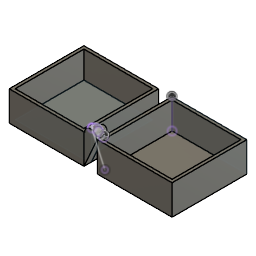
19_20_DAY - Parametric Box (Autodesk Fusion 360 design; units mm, degrees)
part number: 2026-01-02-10-23-45-080
part number: 2026-01-02-10-51-27-139
part number: 2026-01-02-23-14-10-436
Autodesk Fusion 360 part; units mm, degrees
sketch "Box Bottom" plane through (0, 0, 0) normal (0, 1, 0) x (1, 0, 0) in component "Box Top"
  line L0 (0, 0) -> (50, 0)
  line L1 (50, 0) -> (50, 50)
  line L2 (50, 50) -> (0, 50)
  line L3 (0, 50) -> (0, 0)
  dimension "d3" = 50
  dimension "d4" = 50
  constraint horizontal L0
  constraint vertical L1
  constraint horizontal L2
  constraint vertical L3
  constraint coincident L0.start L3.end
  measures "d3" distance of L0.start L2.end
  measures "d4" distance of L1.end L2.end
extrude "Extrude1" add sketch "Box Bottom" along normal blind 20 makes body 1 in component "Box Top"
shell "Shell1" thickness 2 removed faces 1 at (16.6667, 20, -33.3333) on bodies 1 in component "Box Top"
sketch "Box Bottom (2)" plane through (0, 0, 0) normal (0, 1, 0) x (1, 0, 0) in component "Box Top (1)"
  line L0 (0, 0) -> (50, 0)
  line L1 (50, 0) -> (50, 50)
  line L2 (50, 50) -> (0, 50)
  line L3 (0, 50) -> (0, 0)
  dimension "d3_1" = 50
  dimension "d4_1" = 50
  constraint horizontal L0
  constraint vertical L1
  constraint horizontal L2
  constraint vertical L3
  constraint coincident L0.start L3.end
  measures "d3_1" distance of L0.start L2.end
  measures "d4_1" distance of L1.end L2.end
extrude "Extrude1'" add sketch "Box Bottom (2)" along normal blind 20 separate body makes body 2 in component "Box Top (1)"
shell "Shell1'" thickness 2 removed faces 1 at (16.6667, 20, -33.3333) on bodies 2 in component "Box Top (1)"
sketch "Sketch1" plane through (0, 0, 0) normal (0, 0, 1) x (1, 0, 0)
  line L0 (-59, 0) -> (-9, 0)
  line L1 (-9, 0) -> (-9, 20)
  line L2 (-9, 20) -> (-59, 20)
  line L3 (-59, 20) -> (-59, 0)
  line L4 (-9, 20) -> (-4.5, 20)
  circle A0 centre (-4.5, 20) radius 4
  line L5 (-9, 0) -> (-0.8439, 18.3774)
  dimension "d16" = 4.5
  dimension "d17" = 8
  constraint coincident L1.end L2.start
  constraint perpendicular L1 L4
  constraint coincident L4.end A0.centre
  constraint coincident L0.end L1.start
  constraint coincident A0 L5.end
  constraint tangent A0 L5
  measures "d16" distance of L1.end L4.end
  measures "d17" diameter of A0
extrude "Extrude1''" add sketch "Sketch1" against normal blind 5 separate body contours L1 L4 A0 L5 | A0 makes body 3
sketch "Sketch2" plane through (0, 0, -5) normal (0, 0, -1) x (-1, 0, 0)
  line L0 (9, 0) -> (9, 20)
  line L1 (9, 20) -> (8.5, 20)
  arc A0 (8.5, 20) -> (0.8439, 18.3774) centre (4.5, 20) ccw
  line L2 (0.8439, 18.3774) -> (9, 0)
  arc A1 (8.5, 20) -> (0.8439, 18.3774) centre (4.5, 20) ccw
  circle A2 centre (4.5, 20) radius 2
  dimension "d20" = 4
  constraint concentric A1 A2
  measures "d20" diameter of A2
extrude "Extrude2" add sketch "Sketch2" along normal blind 3.8 contours A2 bodies 3
sketch "Sketch3" plane through (0, 2, 0) normal (0, 1, 0) x (-1, 0, 0)
  line L0 (57, -48) -> (57, -2)
  line L1 (57, -2) -> (11, -2)
  line L2 (11, -2) -> (11, -48)
  line L3 (11, -48) -> (57, -48)
sketch "Sketch4" plane through (0, 0, -5) normal (0, 0, -1) x (-1, 0, 0)
  circle A0 centre (4.5, 20) radius 2
  line L0 (9, 0) -> (9, 20)
  line L1 (9, 20) -> (8.5, 20)
  arc A1 (8.5, 20) -> (0.8439, 18.3774) centre (4.5, 20) ccw
  line L2 (0.8439, 18.3774) -> (9, 0)
  arc A2 (8.5, 20) -> (0.8439, 18.3774) centre (4.5, 20) ccw
  circle A3 centre (4.5, 20) radius 4
  line L3 (0, 20) -> (0.5, 20)
  line L4 (0, 0) -> (8.1561, 18.3774)
  constraint concentric A2 A3
  constraint coincident A2 L3.end
  constraint coincident A3 L3.end
  constraint coincident L4.start origin
  constraint coincident A3 L4.end
  constraint tangent A3 L4
  constraint horizontal L3
sketch "Sketch5" plane through (0, 0, -50) normal (0, 0, -1) x (-1, 0, 0)
  line L0 (-50, 0) -> (0, 0)
  line L1 (0, 0) -> (0, 20)
  line L2 (0, 20) -> (-50, 20)
  line L3 (-50, 20) -> (-50, 0)
  line L4 (0, 0) -> (0, 20)
  line L5 (0.5, 20) -> (0, 20)
  constraint coincident L1.end L2.start
  constraint horizontal L5
component "Box Top" placed x (1, 0, 0) y (0, 1, 0) z (0, 0, 1) at (0, 0, 0)
component "Box Top (1)" placed x (1, 0, 0) y (0, 1, 0) z (0, 0, 1) at (-59, 0, 0)
equation "BoxWidth = 50 mm"
equation "BoxHeight = 40 mm"
equation "d3 = BoxWidth"
equation "d4 = BoxWidth"
equation "d5 = BoxHeight / 2"
equation "WallThickness = 2 mm"
equation "d3_1 = BoxWidth"
equation "d4_1 = BoxWidth"
equation "d5_1 = BoxHeight / 2"
equation "WallThickness_1 = 2 mm"
